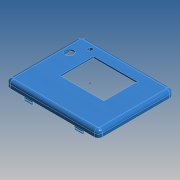
# Autodesk Inventor part: A2_TopCase
Saved by Autodesk Inventor 2020.2 (Build 242310000, 310)
## iProperties
Created: 2021-08-29
Part Number: A2_TopCase
Material: Plastique ABS
Document SubType Name: Modeling
Designer: Samy Francelet
Density: 1.06 g/cm^3
Appearance: Cyan
Author: Samy Francelet
Autodesk Inventor part; units mm, degrees
ref_plane "YZ Plane" through (0, 0, 0) normal (1, 0, 0) x (0, 1, 0)
ref_plane "XZ Plane" through (0, 0, 0) normal (0, 1, 0) x (-1, 0, 0)
ref_plane "XY Plane" through (0, 0, 0) normal (0, 0, 1) x (1, 0, 0)
sketch "Esquisse2" plane through (0, 0, 0) normal (0, 0, 1) x (1, 0, 0)
  line L0 (-78.4497, 0) -> (78.4497, 0) construction
  line L1 (0, -64.4497) -> (0, 64.4497) construction
  line L2 (-50, -45) -> (50, -45)
  line L3 (55, -40) -> (55, 40)
  line L4 (50, 45) -> (-50, 45)
  line L5 (-55, 40) -> (-55, -40)
  line L6 (-55, -45) -> (55, 45) construction
  line L7 (55, -45) -> (-55, 45) construction
  arc A0 (-50, 45) -> (-55, 40) centre (-50, 40) ccw
  arc A1 (-55, -40) -> (-50, -45) centre (-50, -40) ccw
  arc A2 (50, -45) -> (55, -40) centre (50, -40) ccw
  arc A3 (55, 40) -> (50, 45) centre (50, 40) ccw
  point P0 (0, 0)
  dimension "d0" = 110
  dimension "d1" = 90
  dimension "d2" = 5
  constraints: 12 end point, 8 point on circle, 8 point on line, 8 tangent, 4 centre point, 3 equal radius, 2 midpoint, 2 parallel, 1 horizontal, 1 perpendicular
  measures "d0" distance of L7.end L6.end
  measures "d1" distance of L6.end L7.start
  measures "d2" radius of A0
extrude "Extrusion1" add sketch "Esquisse2" along normal blind 8
fillet "Congé1" radius 4 8 edges at (53.5355, -43.5355, 8) (55, 0, 8) (53.5355, 43.5355, 8) (0, 45, 8) (-53.5355, 43.5355, 8) (-55, 0, 8) (-53.5355, -43.5355, 8) (0, -45, 8)
sketch "Esquisse3" plane through (0, 0, 8) normal (0, 0, 1) x (1, 0, 0)
  line L0 (-83, 0) -> (78, 0) construction
  line L1 (0, -64) -> (0, 69) construction
  line L2 (50, 45) -> (-50, 45) construction
  line L3 (-55, 40) -> (-55, -40) construction
  line L4 (-55, 45) -> (-26, 45) construction
  line L5 (-26, 45) -> (-26, 30) construction
  line L6 (-26, 30) -> (-55, 30) construction
  line L7 (-55, 30) -> (-55, 45) construction
  line L8 (-26, 30) -> (26.5, 30)
  line L9 (26.5, 30) -> (26.5, -10)
  line L10 (26.5, -10) -> (-26, -10)
  line L11 (-26, -10) -> (-26, 30)
  point P0 (0, 0)
  dimension "d6" = 29
  dimension "d7" = 15
  dimension "d8" = 52.5
  dimension "d9" = 40
  constraints: 16 end point, 4 parallel, 2 collinear, 2 horizontal, 2 perpendicular
  measures "d6" distance of L5.end L6.end
  measures "d7" distance of L4.end L5.end
  measures "d8" distance of L9.end L10.end
  measures "d9" distance of L8.end L9.end
extrude "Extrusion2" cut sketch "Esquisse3" against normal through all
sketch "Esquisse4" plane through (0, 0, 0) normal (0, 0, -1) x (-1, 0, 0)
  line L0 (0, -71.6569) -> (0, 72.6924) construction
  line L1 (86.6924, 0) -> (-85.6569, 0) construction
  line L2 (-50.5, -42.5) -> (50.5, -42.5)
  line L3 (52.5, -40.5) -> (52.5, 40.5)
  line L4 (50.5, 42.5) -> (-50.5, 42.5)
  line L5 (-52.5, 40.5) -> (-52.5, -40.5)
  line L6 (-52.5, -42.5) -> (52.5, 42.5) construction
  line L7 (52.5, -42.5) -> (-52.5, 42.5) construction
  arc A0 (-50.5, 42.5) -> (-52.5, 40.5) centre (-50.5, 40.5) ccw
  arc A1 (-52.5, -40.5) -> (-50.5, -42.5) centre (-50.5, -40.5) ccw
  arc A2 (50.5, -42.5) -> (52.5, -40.5) centre (50.5, -40.5) ccw
  arc A3 (52.5, 40.5) -> (50.5, 42.5) centre (50.5, 40.5) ccw
  line L8 (-26.5, -10) -> (-26.5, 30) construction
  line L9 (-26.5, 30) -> (26, 30) construction
  line L10 (26, 30) -> (26, -10) construction
  line L11 (26, -10) -> (-26.5, -10) construction
  arc A4 (50, -45) -> (55, -40) centre (50, -40) ccw construction
  line L12 (55, 40) -> (55, -40) construction
  arc A5 (55, 40) -> (50, 45) centre (50, 40) ccw construction
  line L13 (-50, 45) -> (50, 45) construction
  arc A6 (-50, 45) -> (-55, 40) centre (-50, 40) ccw construction
  line L14 (-55, -40) -> (-55, 40) construction
  arc A7 (-55, -40) -> (-50, -45) centre (-50, -40) ccw construction
  line L15 (50, -45) -> (-50, -45) construction
  line L16 (55, 40) -> (55, -40) construction
  line L17 (-50, 45) -> (50, 45) construction
  point P0 (0, 0)
  dimension "d12" = 105
  dimension "d13" = 85
  dimension "d14" = 2
  constraints: 12 end point, 8 point on circle, 8 point on line, 8 tangent, 4 centre point, 3 equal radius, 2 midpoint, 2 parallel, 1 horizontal, 1 perpendicular
  measures "d12" distance of L7.end L6.end
  measures "d13" distance of L6.end L7.start
  measures "d14" radius of A0
extrude "Extrusion3" cut sketch "Esquisse4" against normal blind 6
sketch "Esquisse5" plane through (0, 0, 0) normal (0, 0, -1) x (-1, 0, 0)
  line L0 (0, -71.6569) -> (0, 72.6924) construction
  line L1 (85.6569, 0) -> (-86.6924, 0) construction
  line L2 (-52.5, -40.5) -> (-52.5, 40.5) construction
  arc A0 (-50.5, 42.5) -> (-52.5, 40.5) centre (-50.5, 40.5) ccw construction
  line L3 (-50.5, 42.5) -> (50.5, 42.5) construction
  arc A1 (52.5, 40.5) -> (50.5, 42.5) centre (50.5, 40.5) ccw construction
  line L4 (52.5, 40.5) -> (52.5, -40.5) construction
  arc A2 (50.5, -42.5) -> (52.5, -40.5) centre (50.5, -40.5) ccw construction
  line L5 (50.5, -42.5) -> (-50.5, -42.5) construction
  arc A3 (-52.5, -40.5) -> (-50.5, -42.5) centre (-50.5, -40.5) ccw construction
  arc A4 (50, -45) -> (55, -40) centre (50, -40) ccw construction
  line L6 (55, 40) -> (55, -40) construction
  arc A5 (55, 40) -> (50, 45) centre (50, 40) ccw construction
  line L7 (-50, 45) -> (50, 45) construction
  arc A6 (-50, 45) -> (-55, 40) centre (-50, 40) ccw construction
  line L8 (-55, -40) -> (-55, 40) construction
  arc A7 (-55, -40) -> (-50, -45) centre (-50, -40) ccw construction
  line L9 (50, -45) -> (-50, -45) construction
  line L10 (-55, 45) -> (-35, 45) construction
  line L11 (-35, 45) -> (-35, 42.5) construction
  line L12 (-35, 42.5) -> (-55, 42.5) construction
  line L13 (-55, 42.5) -> (-55, 45) construction
  line L14 (-55, -40) -> (-55, 40) construction
  line L15 (-50, 45) -> (50, 45) construction
  line L16 (-35, 42.5) -> (-25, 42.5)
  line L17 (-25, 42.5) -> (-25, 43.5)
  line L18 (-25, 43.5) -> (-35, 43.5)
  line L19 (-35, 43.5) -> (-35, 42.5)
  point P0 (0, 0)
  dimension "d17" = 20
  dimension "d18" = 2.5
  dimension "d19" = 10
  dimension "d20" = 1
  constraints: 16 end point, 4 parallel, 2 collinear, 2 horizontal, 2 perpendicular
  measures "d17" distance of L11.end L12.end
  measures "d18" distance of L10.end L11.end
  measures "d19" distance of L18.end L17.end
  measures "d20" distance of L17.end L16.end
extrude "Extrusion4" add sketch "Esquisse5" along normal blind 6
sketch "Esquisse6" plane through (25, 43.5, 0) normal (0, 1, 0) x (1, 0, 0)
  line L0 (10, 0) -> (0, 0) construction
  line L1 (10, 0) -> (10, 6) construction
  line L2 (0, 6) -> (10, 6) construction
  line L3 (0, 0) -> (0, 6) construction
  line L4 (0, 6) -> (10, 6)
  line L5 (10, 6) -> (10, 3)
  line L6 (10, 3) -> (0, 3)
  line L7 (0, 3) -> (0, 6)
  point P0 (-25, 0)
  dimension "d23" = 3
  constraints: 8 end point, 2 parallel, 1 horizontal, 1 midpoint, 1 perpendicular
  measures "d23" distance of L4.end L5.end
extrude "Extrusion5" add sketch "Esquisse6" along normal blind 0.5
mirror "Symétrie1" about plane through (0, 0, 0) normal (1, 0, 0) of "Extrusion4", "Extrusion5"
mirror "Symétrie2" about plane through (0, 0, 0) normal (0, 1, 0) of "Extrusion4", "Extrusion5", "Symétrie1"
chamfer "Chanfrein1" distance 2.5 angle 25 1 edges at (30, 44, -6) measured on face at (30, 44, -5.5)
sketch "Esquisse9" plane through (0, 0, 6) normal (0, 0, -1) x (-1, 0, 0)
  line L0 (35, -42.5) -> (35, -43.5) construction
  line L1 (25, -43.5) -> (25, -42.5) construction
  line L2 (-25, -42.5) -> (-25, -43.5) construction
  line L3 (-35, -43.5) -> (-35, -42.5) construction
  line L4 (25, 42.5) -> (25, 43.5) construction
  line L5 (35, 43.5) -> (35, 42.5) construction
  line L6 (-35, 42.5) -> (-35, 43.5) construction
  line L7 (-25, 43.5) -> (-25, 42.5) construction
  arc A0 (52.5, 40.5) -> (50.5, 42.5) centre (50.5, 40.5) ccw construction
  line L8 (52.5, 40.5) -> (52.5, -40.5) construction
  arc A1 (50.5, -42.5) -> (52.5, -40.5) centre (50.5, -40.5) ccw construction
  line L9 (50.5, -42.5) -> (35, -42.5) construction
  arc A2 (-52.5, -40.5) -> (-50.5, -42.5) centre (-50.5, -40.5) ccw construction
  line L10 (-52.5, -40.5) -> (-52.5, 40.5) construction
  arc A3 (-50.5, 42.5) -> (-52.5, 40.5) centre (-50.5, 40.5) ccw construction
  line L11 (-50.5, 42.5) -> (-35, 42.5) construction
  arc A4 (50, -45) -> (55, -40) centre (50, -40) ccw construction
  line L12 (55, 40) -> (55, -40) construction
  arc A5 (55, 40) -> (50, 45) centre (50, 40) ccw construction
  line L13 (-50, 45) -> (50, 45) construction
  arc A6 (-50, 45) -> (-55, 40) centre (-50, 40) ccw construction
  line L14 (-55, -40) -> (-55, 40) construction
  arc A7 (-55, -40) -> (-50, -45) centre (-50, -40) ccw construction
  line L15 (50, -45) -> (-50, -45) construction
  line L16 (55, 40) -> (55, -40) construction
  line L17 (-50, 45) -> (50, 45) construction
  circle A8 centre (35, 35) radius 4
  line L18 (78.4497, 0) -> (-78.4497, 0) construction
  line L19 (0, -64.4497) -> (0, 64.4497) construction
  line L20 (0, 0) -> (35, 0) construction
  line L21 (35, 0) -> (35, 35) construction
  line L22 (35, 35) -> (0, 35) construction
  line L23 (0, 35) -> (0, 0) construction
  line L24 (35, -43.5) -> (25, -43.5) projected
  line L25 (-25, -43.5) -> (-35, -43.5) projected
  line L26 (25, 43.5) -> (35, 43.5) projected
  line L27 (-35, 43.5) -> (-25, 43.5) projected
  line L28 (25, -42.5) -> (-25, -42.5) projected
  line L29 (-35, -42.5) -> (-50.5, -42.5) projected
  line L30 (-25, 42.5) -> (25, 42.5) projected
  line L31 (35, 42.5) -> (50.5, 42.5) projected
  dimension "d49" = 8
  dimension "d52" = 35
  dimension "d53" = 35
  constraints: 8 end point, 2 parallel, 1 centre point, 1 coincident, 1 horizontal, 1 perpendicular
  measures "d49" diameter of A8
  measures "d52" distance of L21.end L22.end
  measures "d53" distance of L20.end L21.end
extrude "Extrusion7" add sketch "Esquisse9" along normal blind 4
sketch "Esquisse7" plane through (0, 0, 8) normal (0, 0, 1) x (1, 0, 0)
  circle A0 centre (-44, 19.5) radius 5
  circle A1 centre (-35, 35) radius 2.7
  line L0 (0, 0) -> (-35, 0) construction
  line L1 (-35, 0) -> (-35, 35) construction
  line L2 (-35, 35) -> (0, 35) construction
  line L3 (0, 35) -> (0, 0) construction
  line L4 (-35, 35) -> (-37.15, 35) construction
  line L5 (-37.15, 33.3668) -> (-37.15, 36.6332)
  line L6 (-32.85, 33.3668) -> (-32.85, 36.6332)
  line L7 (0, 0) -> (-44, 0) construction
  line L8 (-44, 0) -> (-44, 19.5) construction
  line L9 (-44, 19.5) -> (0, 19.5) construction
  line L10 (0, 19.5) -> (0, 0) construction
  dimension "d34" = 10
  dimension "d39" = 5.4
  dimension "d54" = 35
  dimension "d55" = 35
  dimension "d56" = 2.15
  dimension "d57" = 44
  dimension "d58" = 19.5
  constraints: 22 end point, 4 parallel, 3 horizontal, 2 centre point, 2 coincident, 2 perpendicular, 2 point on circle, 2 symmetric about line, 1 midpoint, 1 vertical
  measures "d34" diameter of A0
  measures "d39" diameter of A1
  measures "d54" distance of L1.end L2.end
  measures "d55" distance of L0.end L1.end
  measures "d56" distance of L1.end L4.end
  measures "d57" distance of L8.end L9.end
  measures "d58" distance of L7.end L8.end
extrude "Extrusion6" cut sketch "Esquisse7" against normal through all contours A0 | L6 A1 L5
sketch "Esquisse11" plane through (0, 0, 8) normal (0, 0, 1) x (1, 0, 0)
  point P0 (0, 0)
chamfer "Chanfrein3" distance 2.5 angle 25 1 edges at (-30, 44, -6) measured on face at (-30, 44, -5.5)
chamfer "Chanfrein4" distance 2.5 angle 25 1 edges at (-30, -44, -6) measured on face at (-30, -44, -5.5)
chamfer "Chanfrein5" distance 2.5 angle 25 1 edges at (30, -44, -6) measured on face at (30, -44, -5.5)
